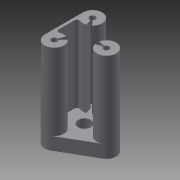
# Autodesk Inventor part: RailGuide
Saved by Autodesk Inventor 2014 (Build 180170000, 170)
## iProperties
Created: 2016-01-26
Part Number: RailGuide
Material: Generic
Document SubType Name: Modeling
Designer: Justin B
Density: 1 g/cm^3
Appearance: Default
Author: Justin B
Autodesk Inventor part; units mm, degrees
ref_plane "YZ Plane" through (0, 0, 0) normal (1, 0, 0) x (0, 1, 0)
ref_plane "XZ Plane" through (0, 0, 0) normal (0, 1, 0) x (-1, 0, 0)
ref_plane "XY Plane" through (0, 0, 0) normal (0, 0, 1) x (1, 0, 0)
sketch "Sketch1" plane through (0, 0, 0) normal (0, 0, 1) x (1, 0, 0)
  circle A0 centre (0, 0) radius 1.5 projected
  circle A1 centre (-8.6603, 15) radius 2.25 projected
  circle A2 centre (17.3205, 0) radius 2.25 projected
  circle A3 centre (-8.6603, -15) radius 2.25 projected
  line L0 (-16.1603, 15) -> (-16.1603, -15) projected
  arc A4 (-16.1603, -15) -> (-4.9103, -21.4952) centre (-8.6603, -15) ccw projected
  line L1 (-4.9103, -21.4952) -> (21.0705, -6.4952) projected
  arc A5 (21.0705, -6.4952) -> (21.0705, 6.4952) centre (17.3205, 0) ccw projected
  line L2 (21.0705, 6.4952) -> (-4.9103, 21.4952) projected
  arc A6 (-4.9103, 21.4952) -> (-16.1603, 15) centre (-8.6603, 15) ccw projected
  point P0 (0, 0)
extrude "Extrusion1" add sketch "Sketch1" along normal blind 10 contours A0 | A1 | A2 | A3 | A6 L2 A5 L1 A4 L0
sketch "Sketch2" plane through (0, 0, 0) normal (0, 0, -1) x (-1, 0, 0)
  arc A0 (16.1603, 15) -> (4.9103, 21.4952) centre (8.6603, 15) ccw projected
  arc A1 (-21.0705, 6.4952) -> (-21.0705, -6.4952) centre (-17.3205, 0) ccw projected
  arc A2 (4.9103, -21.4952) -> (16.1603, -15) centre (8.6603, -15) ccw projected
hole "Hole1" at (17.3205, 0, 0) at (-8.6603, 15, 0) at (-8.6603, -15, 0) direction (0, 0, 1) diameter 4.5 depth 4.25
sketch "Sketch3" plane through (0, 0, 10) normal (0, 0, 1) x (1, 0, 0)
  arc A0 (-16.1603, -15) -> (-4.9103, -21.4952) centre (-8.6603, -15) ccw projected
  arc A1 (21.0705, -6.4952) -> (21.0705, 6.4952) centre (17.3205, 0) ccw projected
  arc A2 (-4.9103, 21.4952) -> (-16.1603, 15) centre (-8.6603, 15) ccw projected
  circle A3 centre (-8.6603, 15) radius 7.5
  circle A4 centre (17.3205, 0) radius 7.5
  circle A5 centre (-8.6603, -15) radius 7.5
  constraints: 3 centre point, 3 coincident, 3 concentric
extrude "Extrusion2" add sketch "Sketch3" along normal blind 60
sketch "Sketch4" plane through (-8.6603, -15, 70) normal (0, 0, 1) x (1, 0, 0)
  circle A0 centre (0, 0) radius 7.5 projected
  arc A1 (29.7308, 21.4952) -> (29.7308, 8.5048) centre (25.9808, 15) ccw projected
  arc A2 (-7.5, 30) -> (3.75, 36.4952) centre (0, 30) ccw projected
  point P0 (8.6603, 15)
hole "Hole2" at (-8.6603, 15, 70) at (17.3205, 0, 70) at (-8.6603, -15, 70) direction (0, 0, -1) diameter 4.5 depth 60
sketch "Sketch5" plane through (0, 0, 10) normal (0, 0, 1) x (1, 0, 0)
  arc A0 (21.0705, 6.4952) -> (21.0705, -6.4952) centre (17.3205, 0) ccw projected
  arc A1 (-16.1603, 15) -> (-4.9103, 21.4952) centre (-8.6603, 15) ccw projected
  arc A2 (-4.9103, -21.4952) -> (-16.1603, -15) centre (-8.6603, -15) ccw projected
  line L0 (-4.9103, -21.4952) -> (21.0705, -6.4952) projected
  circle A3 centre (0, 0) radius 1.5 projected
  line L1 (-4, 0) -> (2, -3.4641) construction
  line L2 (2, -3.4641) -> (2, 3.4641) construction
  line L3 (2, 3.4641) -> (-4, 0) construction
  line L4 (-8.6603, 15) -> (0, 0) construction
  line L5 (-8.6603, -15) -> (-4, 0)
  line L6 (-8.6603, 15) -> (-4, 0)
  line L7 (-8.6603, 15) -> (2, 3.4641)
  line L8 (2, 3.4641) -> (17.3205, 0)
  line L9 (17.3205, 0) -> (2, -3.4641)
  line L10 (2, -3.4641) -> (-8.6603, -15)
  dimension "d18" = 4
  dimension "d19" = 4
  dimension "d20" = 4
  constraints: 20 end point, 2 equal length, 2 perpendicular
  measures "d18" distance of L4.end L1.end
  measures "d19" distance of L2.end L4.end
  measures "d20" distance of L1.start L4.end
extrude "Extrusion3" cut sketch "Sketch5" along normal blind 60 contours L8 L9 A0 | A0 L9 L10 A2 L5 L6 A1 L7 L8 | A1 L6 L7 | L10 L5 A2
sketch "Sketch6" plane through (0, 0, 10) normal (0, 0, 1) x (1, 0, 0)
  arc A0 (-16.1603, 15) -> (-6.435, 7.8377) centre (-8.6603, 15) ccw projected
  line L0 (-16.1603, 15) -> (-16.1603, -15) projected
  arc A1 (-6.435, -7.8377) -> (-16.1603, -15) centre (-8.6603, -15) ccw projected
  line L1 (-14.1603, -9.901) -> (-14.1603, 9.901)
  dimension "d26" = 2
  constraints: 2 end point, 2 point on circle, 1 parallel
  measures "d26" distance between parallel lines of L0 L1
extrude "Extrusion4" add sketch "Sketch6" along normal blind 60
sketch "Sketch8" plane through (0, 0, 10) normal (0, 0, 1) x (1, 0, 0)
  circle A0 centre (0, 0) radius 5
  dimension "d41" = 10
  constraints: 1 centre point, 1 coincident
  measures "d41" diameter of A0
hole "Hole3" at (0, 0, 10) direction (0, 0, -1) diameter 10 end through all
pattern_circular "Circular Pattern1" count 3 over 360 about axis through (0, 0, -82.76) along (0, 0, 1) of "Extrusion4"
sketch "Sketch7" plane through (-4.9103, 21.4952, 70) normal (0.5, 0.8660254, 0) x (0.8660254, -0.5, 0)
  line L0 (30, 70) -> (0, 70) projected
  line L1 (0, 70) -> (0, 60) projected
  line L2 (30, 0) -> (0, 0) projected
  line L3 (15.4514, 50) -> (15.4514, 20) construction
  line L4 (9.4514, 50) -> (9.4514, 20)
  line L5 (21.4514, 20) -> (21.4514, 50)
  arc A0 (21.4514, 50) -> (9.4514, 50) centre (15.4514, 50) ccw
  arc A1 (9.4514, 20) -> (21.4514, 20) centre (15.4514, 20) ccw
  line L6 (30, 70) -> (0, 70) projected
  line L7 (0, 70) -> (0, 0) projected
  line L8 (30, 70) -> (30, 0) projected
  line L9 (30, 0) -> (0, 0) projected
  point P0 (15, 70)
  point P1 (15.4514, 35)
  dimension "d32" = 20
  dimension "d33" = 20
  dimension "d34" = 6
  constraints: 8 end point, 4 point on circle, 4 tangent, 2 centre point, 2 parallel, 1 midpoint
  measures "d32" distance from line of L2 L5.start
  measures "d33" distance from line of L0 L5.end
  measures "d34" radius of A0
extrude "Extrusion5" cut sketch "Sketch7" against normal blind 4 contours A0 L5 A1 L4
pattern_circular "Circular Pattern2" count 3 over 360 about axis through (0, 0, -82.76) along (0, 0, 1) of "Extrusion5"
fillet "Fillet1" radius 2 6 edges at (-14.1603, 9.901, 40) (-14.1603, -9.901, 40) (-1.4944, -17.2136, 40) (-1.4944, 17.2136, 40) (15.6546, 7.3126, 40) (15.6546, -7.3126, 40)
equation "\"d19\" = d18"
equation "\"d20\" = d18"
equation "\"d33\" = d32"
body "Solid1"
